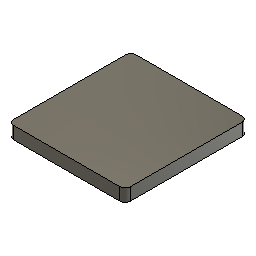
pzt-element-tray (Autodesk Fusion 360 design; units mm, degrees)
Autodesk Fusion 360 part; units mm, degrees
note: some values were not read from the file. Set by a fixed rule: the direction of a hole.
sketch "Sketch1" plane through (0, 0, 0) normal (0, 1, 0) x (1, 0, 0)
  circle A0 centre (0, 0) radius 1.5 construction
  circle A1 centre (5.5, 0) radius 1.5 construction
  circle A2 centre (11, 0) radius 1.5 construction
  circle A3 centre (16.5, 0) radius 1.5 construction
  circle A4 centre (22, 0) radius 1.5 construction
  circle A5 centre (27.5, 0) radius 1.5 construction
  circle A6 centre (33, 0) radius 1.5 construction
  circle A7 centre (38.5, 0) radius 1.5 construction
  circle A8 centre (44, 0) radius 1.5 construction
  circle A9 centre (49.5, 0) radius 1.5 construction
  circle A10 centre (55, 0) radius 1.5 construction
  circle A11 centre (60.5, 0) radius 1.5 construction
  circle A12 centre (0, 5.5) radius 1.5 construction
  circle A13 centre (5.5, 5.5) radius 1.5 construction
  circle A14 centre (11, 5.5) radius 1.5 construction
  circle A15 centre (16.5, 5.5) radius 1.5 construction
  circle A16 centre (22, 5.5) radius 1.5 construction
  circle A17 centre (27.5, 5.5) radius 1.5 construction
  circle A18 centre (33, 5.5) radius 1.5 construction
  circle A19 centre (38.5, 5.5) radius 1.5 construction
  circle A20 centre (44, 5.5) radius 1.5 construction
  circle A21 centre (49.5, 5.5) radius 1.5 construction
  circle A22 centre (55, 5.5) radius 1.5 construction
  circle A23 centre (60.5, 5.5) radius 1.5 construction
  circle A24 centre (0, 11) radius 1.5 construction
  circle A25 centre (5.5, 11) radius 1.5 construction
  circle A26 centre (11, 11) radius 1.5 construction
  circle A27 centre (16.5, 11) radius 1.5 construction
  circle A28 centre (22, 11) radius 1.5 construction
  circle A29 centre (27.5, 11) radius 1.5 construction
  circle A30 centre (33, 11) radius 1.5 construction
  circle A31 centre (38.5, 11) radius 1.5 construction
  circle A32 centre (44, 11) radius 1.5 construction
  circle A33 centre (49.5, 11) radius 1.5 construction
  circle A34 centre (55, 11) radius 1.5 construction
  circle A35 centre (60.5, 11) radius 1.5 construction
  circle A36 centre (0, 16.5) radius 1.5 construction
  circle A37 centre (5.5, 16.5) radius 1.5 construction
  circle A38 centre (11, 16.5) radius 1.5 construction
  circle A39 centre (16.5, 16.5) radius 1.5 construction
  circle A40 centre (22, 16.5) radius 1.5 construction
  circle A41 centre (27.5, 16.5) radius 1.5 construction
  circle A42 centre (33, 16.5) radius 1.5 construction
  circle A43 centre (38.5, 16.5) radius 1.5 construction
  circle A44 centre (44, 16.5) radius 1.5 construction
  circle A45 centre (49.5, 16.5) radius 1.5 construction
  circle A46 centre (55, 16.5) radius 1.5 construction
  circle A47 centre (60.5, 16.5) radius 1.5 construction
  line L0 (-14.5, -14.5) -> (97, -14.5)
  line L1 (97, -14.5) -> (97, 102.5)
  line L2 (97, 102.5) -> (-14.5, 102.5)
  line L3 (-14.5, 102.5) -> (-14.5, -14.5)
  line L4 (0, 0) -> (0, -1.5) construction
  line L5 (0, 0) -> (-1.5, 0) construction
  line L6 (-1.5, 0) -> (-14.5, 0) construction
  line L7 (0, 0) -> (-14.5, -14.5) construction
  line L8 (0, -1.5) -> (0, -14.5) construction
  line L9 (82.5, 88) -> (82.5, 0) construction
  line L10 (82.5, 0) -> (0, 0) construction
  line L11 (82.5, 88) -> (97, 102.5) construction
  circle A48 centre (66, 0) radius 1.5 construction
  circle A49 centre (71.5, 0) radius 1.5 construction
  circle A50 centre (77, 0) radius 1.5 construction
  circle A51 centre (82.5, 0) radius 1.5 construction
  circle A52 centre (66, 5.5) radius 1.5 construction
  circle A53 centre (71.5, 5.5) radius 1.5 construction
  circle A54 centre (77, 5.5) radius 1.5 construction
  circle A55 centre (82.5, 5.5) radius 1.5 construction
  circle A56 centre (66, 11) radius 1.5 construction
  circle A57 centre (71.5, 11) radius 1.5 construction
  circle A58 centre (77, 11) radius 1.5 construction
  circle A59 centre (82.5, 11) radius 1.5 construction
  circle A60 centre (66, 16.5) radius 1.5 construction
  circle A61 centre (71.5, 16.5) radius 1.5 construction
  circle A62 centre (77, 16.5) radius 1.5 construction
  circle A63 centre (82.5, 16.5) radius 1.5 construction
  circle A64 centre (0, 22) radius 1.5 construction
  circle A65 centre (5.5, 22) radius 1.5 construction
  circle A66 centre (11, 22) radius 1.5 construction
  circle A67 centre (16.5, 22) radius 1.5 construction
  circle A68 centre (22, 22) radius 1.5 construction
  circle A69 centre (27.5, 22) radius 1.5 construction
  circle A70 centre (33, 22) radius 1.5 construction
  circle A71 centre (38.5, 22) radius 1.5 construction
  circle A72 centre (44, 22) radius 1.5 construction
  circle A73 centre (49.5, 22) radius 1.5 construction
  circle A74 centre (55, 22) radius 1.5 construction
  circle A75 centre (60.5, 22) radius 1.5 construction
  circle A76 centre (66, 22) radius 1.5 construction
  circle A77 centre (71.5, 22) radius 1.5 construction
  circle A78 centre (77, 22) radius 1.5 construction
  circle A79 centre (82.5, 22) radius 1.5 construction
  circle A80 centre (0, 27.5) radius 1.5 construction
  circle A81 centre (5.5, 27.5) radius 1.5 construction
  circle A82 centre (11, 27.5) radius 1.5 construction
  circle A83 centre (16.5, 27.5) radius 1.5 construction
  circle A84 centre (22, 27.5) radius 1.5 construction
  circle A85 centre (27.5, 27.5) radius 1.5 construction
  circle A86 centre (33, 27.5) radius 1.5 construction
  circle A87 centre (38.5, 27.5) radius 1.5 construction
  circle A88 centre (44, 27.5) radius 1.5 construction
  circle A89 centre (49.5, 27.5) radius 1.5 construction
  circle A90 centre (55, 27.5) radius 1.5 construction
  circle A91 centre (60.5, 27.5) radius 1.5 construction
  circle A92 centre (66, 27.5) radius 1.5 construction
  circle A93 centre (71.5, 27.5) radius 1.5 construction
  circle A94 centre (77, 27.5) radius 1.5 construction
  circle A95 centre (82.5, 27.5) radius 1.5 construction
  circle A96 centre (0, 33) radius 1.5 construction
  circle A97 centre (5.5, 33) radius 1.5 construction
  circle A98 centre (11, 33) radius 1.5 construction
  circle A99 centre (16.5, 33) radius 1.5 construction
  circle A100 centre (22, 33) radius 1.5 construction
  circle A101 centre (27.5, 33) radius 1.5 construction
  circle A102 centre (33, 33) radius 1.5 construction
  circle A103 centre (38.5, 33) radius 1.5 construction
  circle A104 centre (44, 33) radius 1.5 construction
  circle A105 centre (49.5, 33) radius 1.5 construction
  circle A106 centre (55, 33) radius 1.5 construction
  circle A107 centre (60.5, 33) radius 1.5 construction
  circle A108 centre (66, 33) radius 1.5 construction
  circle A109 centre (71.5, 33) radius 1.5 construction
  circle A110 centre (77, 33) radius 1.5 construction
  circle A111 centre (82.5, 33) radius 1.5 construction
  circle A112 centre (0, 38.5) radius 1.5 construction
  circle A113 centre (5.5, 38.5) radius 1.5 construction
  circle A114 centre (11, 38.5) radius 1.5 construction
  circle A115 centre (16.5, 38.5) radius 1.5 construction
  circle A116 centre (22, 38.5) radius 1.5 construction
  circle A117 centre (27.5, 38.5) radius 1.5 construction
  circle A118 centre (33, 38.5) radius 1.5 construction
  circle A119 centre (38.5, 38.5) radius 1.5 construction
  circle A120 centre (44, 38.5) radius 1.5 construction
  circle A121 centre (49.5, 38.5) radius 1.5 construction
  circle A122 centre (55, 38.5) radius 1.5 construction
  circle A123 centre (60.5, 38.5) radius 1.5 construction
  circle A124 centre (66, 38.5) radius 1.5 construction
  circle A125 centre (71.5, 38.5) radius 1.5 construction
  circle A126 centre (77, 38.5) radius 1.5 construction
  circle A127 centre (82.5, 38.5) radius 1.5 construction
  circle A128 centre (0, 44) radius 1.5 construction
  circle A129 centre (5.5, 44) radius 1.5 construction
  circle A130 centre (11, 44) radius 1.5 construction
  circle A131 centre (16.5, 44) radius 1.5 construction
  circle A132 centre (22, 44) radius 1.5 construction
  circle A133 centre (27.5, 44) radius 1.5 construction
  circle A134 centre (33, 44) radius 1.5 construction
  circle A135 centre (38.5, 44) radius 1.5 construction
  circle A136 centre (44, 44) radius 1.5 construction
  circle A137 centre (49.5, 44) radius 1.5 construction
  circle A138 centre (55, 44) radius 1.5 construction
  circle A139 centre (60.5, 44) radius 1.5 construction
  circle A140 centre (66, 44) radius 1.5 construction
  circle A141 centre (71.5, 44) radius 1.5 construction
  circle A142 centre (77, 44) radius 1.5 construction
  circle A143 centre (82.5, 44) radius 1.5 construction
  circle A144 centre (0, 49.5) radius 1.5 construction
  circle A145 centre (5.5, 49.5) radius 1.5 construction
  circle A146 centre (11, 49.5) radius 1.5 construction
  circle A147 centre (16.5, 49.5) radius 1.5 construction
  circle A148 centre (22, 49.5) radius 1.5 construction
  circle A149 centre (27.5, 49.5) radius 1.5 construction
  circle A150 centre (33, 49.5) radius 1.5 construction
  circle A151 centre (38.5, 49.5) radius 1.5 construction
  circle A152 centre (44, 49.5) radius 1.5 construction
  circle A153 centre (49.5, 49.5) radius 1.5 construction
  circle A154 centre (55, 49.5) radius 1.5 construction
  circle A155 centre (60.5, 49.5) radius 1.5 construction
  circle A156 centre (66, 49.5) radius 1.5 construction
  circle A157 centre (71.5, 49.5) radius 1.5 construction
  circle A158 centre (77, 49.5) radius 1.5 construction
  circle A159 centre (82.5, 49.5) radius 1.5 construction
  circle A160 centre (0, 55) radius 1.5 construction
  circle A161 centre (5.5, 55) radius 1.5 construction
  circle A162 centre (11, 55) radius 1.5 construction
  circle A163 centre (16.5, 55) radius 1.5 construction
  circle A164 centre (22, 55) radius 1.5 construction
  circle A165 centre (27.5, 55) radius 1.5 construction
  circle A166 centre (33, 55) radius 1.5 construction
  circle A167 centre (38.5, 55) radius 1.5 construction
  circle A168 centre (44, 55) radius 1.5 construction
  circle A169 centre (49.5, 55) radius 1.5 construction
  circle A170 centre (55, 55) radius 1.5 construction
  circle A171 centre (60.5, 55) radius 1.5 construction
  circle A172 centre (66, 55) radius 1.5 construction
  circle A173 centre (71.5, 55) radius 1.5 construction
  circle A174 centre (77, 55) radius 1.5 construction
  circle A175 centre (82.5, 55) radius 1.5 construction
  circle A176 centre (0, 60.5) radius 1.5 construction
  circle A177 centre (5.5, 60.5) radius 1.5 construction
  circle A178 centre (11, 60.5) radius 1.5 construction
  circle A179 centre (16.5, 60.5) radius 1.5 construction
  circle A180 centre (22, 60.5) radius 1.5 construction
  circle A181 centre (27.5, 60.5) radius 1.5 construction
  circle A182 centre (33, 60.5) radius 1.5 construction
  circle A183 centre (38.5, 60.5) radius 1.5 construction
  circle A184 centre (44, 60.5) radius 1.5 construction
  circle A185 centre (49.5, 60.5) radius 1.5 construction
  circle A186 centre (55, 60.5) radius 1.5 construction
  circle A187 centre (60.5, 60.5) radius 1.5 construction
  circle A188 centre (66, 60.5) radius 1.5 construction
  circle A189 centre (71.5, 60.5) radius 1.5 construction
  circle A190 centre (77, 60.5) radius 1.5 construction
  circle A191 centre (82.5, 60.5) radius 1.5 construction
  circle A192 centre (0, 66) radius 1.5 construction
  circle A193 centre (5.5, 66) radius 1.5 construction
  circle A194 centre (11, 66) radius 1.5 construction
  circle A195 centre (16.5, 66) radius 1.5 construction
  circle A196 centre (22, 66) radius 1.5 construction
  circle A197 centre (27.5, 66) radius 1.5 construction
  circle A198 centre (33, 66) radius 1.5 construction
  circle A199 centre (38.5, 66) radius 1.5 construction
  circle A200 centre (44, 66) radius 1.5 construction
  circle A201 centre (49.5, 66) radius 1.5 construction
  circle A202 centre (55, 66) radius 1.5 construction
  circle A203 centre (60.5, 66) radius 1.5 construction
  circle A204 centre (66, 66) radius 1.5 construction
  circle A205 centre (71.5, 66) radius 1.5 construction
  circle A206 centre (77, 66) radius 1.5 construction
  circle A207 centre (82.5, 66) radius 1.5 construction
  circle A208 centre (0, 71.5) radius 1.5 construction
  circle A209 centre (5.5, 71.5) radius 1.5 construction
  circle A210 centre (11, 71.5) radius 1.5 construction
  circle A211 centre (16.5, 71.5) radius 1.5 construction
  circle A212 centre (22, 71.5) radius 1.5 construction
  circle A213 centre (27.5, 71.5) radius 1.5 construction
  circle A214 centre (33, 71.5) radius 1.5 construction
  circle A215 centre (38.5, 71.5) radius 1.5 construction
  circle A216 centre (44, 71.5) radius 1.5 construction
  circle A217 centre (49.5, 71.5) radius 1.5 construction
  circle A218 centre (55, 71.5) radius 1.5 construction
  circle A219 centre (60.5, 71.5) radius 1.5 construction
  circle A220 centre (66, 71.5) radius 1.5 construction
  circle A221 centre (71.5, 71.5) radius 1.5 construction
  circle A222 centre (77, 71.5) radius 1.5 construction
  circle A223 centre (82.5, 71.5) radius 1.5 construction
  circle A224 centre (0, 77) radius 1.5 construction
  circle A225 centre (5.5, 77) radius 1.5 construction
  circle A226 centre (11, 77) radius 1.5 construction
  circle A227 centre (16.5, 77) radius 1.5 construction
  circle A228 centre (22, 77) radius 1.5 construction
  circle A229 centre (27.5, 77) radius 1.5 construction
  circle A230 centre (33, 77) radius 1.5 construction
  circle A231 centre (38.5, 77) radius 1.5 construction
  circle A232 centre (44, 77) radius 1.5 construction
  circle A233 centre (49.5, 77) radius 1.5 construction
  circle A234 centre (55, 77) radius 1.5 construction
  circle A235 centre (60.5, 77) radius 1.5 construction
  circle A236 centre (66, 77) radius 1.5 construction
  circle A237 centre (71.5, 77) radius 1.5 construction
  circle A238 centre (77, 77) radius 1.5 construction
  circle A239 centre (82.5, 77) radius 1.5 construction
  circle A240 centre (0, 82.5) radius 1.5 construction
  circle A241 centre (5.5, 82.5) radius 1.5 construction
  circle A242 centre (11, 82.5) radius 1.5 construction
  circle A243 centre (16.5, 82.5) radius 1.5 construction
  circle A244 centre (22, 82.5) radius 1.5 construction
  circle A245 centre (27.5, 82.5) radius 1.5 construction
  circle A246 centre (33, 82.5) radius 1.5 construction
  circle A247 centre (38.5, 82.5) radius 1.5 construction
  circle A248 centre (44, 82.5) radius 1.5 construction
  circle A249 centre (49.5, 82.5) radius 1.5 construction
  circle A250 centre (55, 82.5) radius 1.5 construction
  circle A251 centre (60.5, 82.5) radius 1.5 construction
  circle A252 centre (66, 82.5) radius 1.5 construction
  circle A253 centre (71.5, 82.5) radius 1.5 construction
  circle A254 centre (77, 82.5) radius 1.5 construction
  circle A255 centre (82.5, 82.5) radius 1.5 construction
  circle A256 centre (0, 88) radius 1.5 construction
  circle A257 centre (5.5, 88) radius 1.5 construction
  circle A258 centre (11, 88) radius 1.5 construction
  circle A259 centre (16.5, 88) radius 1.5 construction
  circle A260 centre (22, 88) radius 1.5 construction
  circle A261 centre (27.5, 88) radius 1.5 construction
  circle A262 centre (33, 88) radius 1.5 construction
  circle A263 centre (38.5, 88) radius 1.5 construction
  circle A264 centre (44, 88) radius 1.5 construction
  circle A265 centre (49.5, 88) radius 1.5 construction
  circle A266 centre (55, 88) radius 1.5 construction
  circle A267 centre (60.5, 88) radius 1.5 construction
  circle A268 centre (66, 88) radius 1.5 construction
  circle A269 centre (71.5, 88) radius 1.5 construction
  circle A270 centre (77, 88) radius 1.5 construction
  circle A271 centre (82.5, 88) radius 1.5 construction
  dimension "d8" = 3
  dimension "d11" = 5.5
  dimension "d12" = 5.5
  dimension "d20" = 13
  dimension "d31" = 82.5
  dimension "d32" = 88
  dimension "d33" = 45
  constraint coincident A0.centre L4.start
  constraint horizontal L0
  constraint vertical L1
  constraint horizontal L2
  constraint vertical L3
  constraint coincident A0 L4.end
  constraint vertical L4
  constraint coincident A0 L5.end
  constraint perpendicular L4 L5
  constraint coincident L3 L6.end
  constraint perpendicular L3 L6
  constraint coincident L0 L8.end
  constraint perpendicular L0 L8
  constraint equal L6 L8
  constraint horizontal L10
  constraint vertical L9
  constraint equal L7 L11
  measures "d8" diameter of A0
  measures "d20" distance of L4.end L8.end
  measures "d31" horizontal distance of L9.end A0.centre
  measures "d32" distance of L9.start L9.end
  measures "d33" angle of L1 L11
extrude "Extrude1" add sketch "Sketch1" along normal blind 9
hole "Hole2" at (0, 0, 0) direction (0, 1, 0) diameter 3 depth 8 tip angle 180
pattern_linear "R-Pattern1" count 17 spacing 5.5 along (0, 0, -1) count 16 spacing 5.5 along (1, 0, 0) of "Hole2"
sketch "Sketch2" plane through (0, 0, 0) normal (0, -1, 0) x (1, 0, 0)
  line L0 (-14.5, 14.5) -> (97, 14.5)
  line L1 (-14.5, -102.5) -> (-14.5, 14.5)
  line L2 (97, -102.5) -> (-14.5, -102.5)
  line L3 (97, 14.5) -> (97, -102.5)
  line L4 (87, -92.5) -> (-4.5, -92.5)
  line L5 (-4.5, -92.5) -> (-4.5, 4.5)
  line L6 (-4.5, 4.5) -> (87, 4.5)
  line L7 (87, 4.5) -> (87, -92.5)
  line L8 (87, -92.5) -> (97, -102.5) construction
  line L9 (87, 4.5) -> (97, 14.5) construction
  line L10 (-4.5, 4.5) -> (-14.5, 14.5) construction
  line L11 (-4.5, -92.5) -> (-14.5, -102.5) construction
  point P0 (-9.5, 9.5)
  point P1 (92, 9.5)
  point P2 (92, -97.5)
  point P3 (-9.5, -97.5)
  dimension "d41" = 10
  constraint coincident L2.start L3.end
  constraint coincident L0.end L3.start
  constraint coincident L0.start L1.end
  constraint coincident L1.start L2.end
  constraint midpoint L10 P0
  constraint midpoint L9 P1
  constraint midpoint L8 P2
  constraint midpoint L11 P3
extrude "Extrude4" add sketch "Sketch2" along normal blind 3
sketch "Sketch6" plane through (0, -3, 0) normal (0, -1, 0) x (1, 0, 0)
  line L0 (-4.5, 4.5) -> (87, 4.5)
  line L1 (87, 4.5) -> (87, -92.5)
  line L2 (87, -92.5) -> (-4.5, -92.5)
  line L3 (-4.5, -92.5) -> (-4.5, 4.5)
  line L4 (97, 14.5) -> (-14.5, 14.5)
  line L5 (-14.5, 14.5) -> (-14.5, -102.5)
  line L6 (-14.5, -102.5) -> (97, -102.5)
  line L7 (97, -102.5) -> (97, 14.5)
  point P0 (-9.5, 9.5)
  point P1 (92, 9.5)
  point P2 (92, -97.5)
  point P3 (-9.5, -97.5)
hole "Hole1" at (-9.5, -3, 9.5) at (92, -3, 9.5) at (92, -3, -97.5) at (-9.5, -3, -97.5) direction (0, 1, 0) diameter 4.1 depth 6 tip angle 180
fillet "Fillet2" radius 5 4 edges at (97, 3, -102.5) (97, 3, 14.5) (-14.5, 3, -102.5) (-14.5, 3, 14.5)
equation "Nrows = 17" comment "User Input"
equation "Ncolumns = 16" comment "User Input"
equation "hole_diameter = 3 mm" comment "User Input"
equation "hole_pitch = 5.5 mm"
equation "hole_depth = pzt_element_length - 2 mm"
equation "border_width = 10 mm"
equation "base_thickness = 1 mm"
equation "d8 = hole_diameter"
equation "d9 = Ncolumns"
equation "d10 = Nrows"
equation "d11 = hole_pitch"
equation "d12 = hole_pitch"
equation "d15 = base_thickness + hole_depth"
equation "border_height = 3 mm"
equation "d20 = border_width + hole_diameter"
equation "M3_insert_diameter = 4.1 mm"
equation "M3_insert_depth = 6 mm"
equation "d26 = M3_insert_depth"
equation "d27 = M3_insert_diameter"
equation "d31 = ( Ncolumns - 1 ) * hole_pitch"
equation "d32 = ( Nrows - 1 ) * hole_pitch"
equation "d34 = hole_depth"
equation "d35 = hole_diameter"
equation "d37 = Nrows"
equation "d38 = Ncolumns"
equation "d39 = hole_pitch"
equation "d40 = hole_pitch"
equation "d41 = border_width"
equation "d42 = border_height"
equation "pzt_element_length = 10 mm" comment "User Input"
named bodies: "PZT Element Tray"
